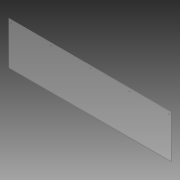
# Autodesk Inventor part: FE-100-001 Main Panel
Saved by Autodesk Inventor 2021 (Build 250183000, 183)
## iProperties
Created: 2021-01-12
Part Number: FE-100-001 Main Panel
Material: Polycarbonate, Clear
Document SubType Name: Modeling
Density: 1.2 g/cm^3
Appearance: Polycarbonate - Clear
Autodesk Inventor part; units mm, degrees
ref_plane "YZ Plane" through (0, 0, 0) normal (1, 0, 0) x (0, 1, 0)
ref_plane "XZ Plane" through (0, 0, 0) normal (0, 1, 0) x (-1, 0, 0)
ref_plane "XY Plane" through (0, 0, 0) normal (0, 0, 1) x (1, 0, 0)
sketch "Sketch1" plane through (0, 0, 0) normal (0, 0, 1) x (1, 0, 0)
  line L0 (-914.4, -241.3) -> (914.4, -241.3)
  line L1 (914.4, -241.3) -> (914.4, 241.3)
  line L2 (914.4, 241.3) -> (-914.4, 241.3)
  line L3 (-914.4, 241.3) -> (-914.4, -241.3)
  line L4 (-914.4, -241.3) -> (914.4, 241.3) construction
  line L5 (914.4, -241.3) -> (-914.4, 241.3) construction
  circle A0 centre (-889, 209.55) radius 4.7625
  circle A1 centre (-444.5, 209.55) radius 4.7625
  circle A2 centre (0, 209.55) radius 4.7625
  circle A3 centre (444.5, 209.55) radius 4.7625
  circle A4 centre (889, 209.55) radius 4.7625
  point P0 (0, 0)
  point P1 (0, 0)
  dimension "d0" = 1828.8
  dimension "d1" = 482.6
  dimension "d2" = 9.525
  dimension "d3" = 31.75
  dimension "d6" = 444.5
  constraints: 12 end point, 5 centre point, 3 midpoint, 2 horizontal, 2 parallel, 1 perpendicular, 1 vertical alignment, 8 other
  measures "d0" distance of L2.end L1.end
  measures "d1" distance of L1.end L0.end
  measures "d2" diameter of A0
  measures "d3" distance from line of A0.centre L2
  measures "d6" distance of A0.centre A1.centre
extrude "Extrusion1" add sketch "Sketch1" along normal blind 6.35
body "Solid1"
